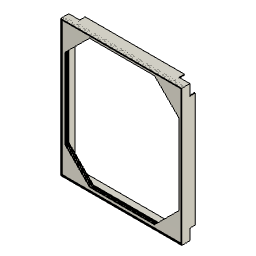
Step4-FaceFrame-4X (Autodesk Fusion 360 design; units mm, degrees)
Autodesk Fusion 360 part; units mm, degrees
note: some values were not read from the file. Set by a fixed rule: which sketch regions a step uses.
sketch "Sketch1" plane through (0, 0, 0) normal (0, 1, 0) x (1, 0, 0)
  line L0 (0, 0) -> (445, 0)
  line L1 (445, 0) -> (445, -500)
  line L2 (445, -500) -> (0, -500)
  line L3 (0, -500) -> (0, 0)
  dimension "d1" = 445
  dimension "d2" = 500
  constraint horizontal L0
  constraint vertical L1
  constraint horizontal L2
  constraint vertical L3
  constraint coincident L0.start L3.end
  measures "d1" distance of L0.start L0.end
  measures "d2" distance of L0.start L2.end
extrude "Extrude1" add sketch "Sketch1" along normal blind 50
ref_plane "WorkPlane1" through (222.5, 0, 250) normal (0, -1, 0) x (-1, 0, 0)
sketch "Sketch2" plane through (222.5, 0, 250) normal (0, -1, 0) x (1, 0, 0)
  line L0 (222.5, 250) -> (119.5, 250)
  line L1 (119.5, 250) -> (119.5, 237)
  line L2 (119.5, 237) -> (222.5, 237)
  line L3 (222.5, 237) -> (222.5, 250)
  line L4 (222.5, 250) -> (209.5, 250)
  line L5 (209.5, 250) -> (209.5, 147)
  line L6 (209.5, 147) -> (222.5, 147)
  line L7 (222.5, 147) -> (222.5, 250)
  line L8 (119.5, 237) -> (209.5, 147)
  line L9 (209.5, 237) -> (119.5, 237)
  line L10 (-222.5, 250) -> (-119.5, 250)
  line L11 (-119.5, 250) -> (-119.5, 237)
  line L12 (-119.5, 237) -> (-222.5, 237)
  line L13 (-222.5, 237) -> (-222.5, 250)
  line L14 (-222.5, 250) -> (-209.5, 250)
  line L15 (-209.5, 250) -> (-209.5, 147)
  line L16 (-209.5, 147) -> (-222.5, 147)
  line L17 (-222.5, 147) -> (-222.5, 250)
  line L18 (-222.5, -250) -> (-119.5, -250)
  line L19 (-119.5, -250) -> (-119.5, -237)
  line L20 (-119.5, -237) -> (-222.5, -237)
  line L21 (-222.5, -237) -> (-222.5, -250)
  line L22 (-222.5, -250) -> (-209.5, -250)
  line L23 (-209.5, -250) -> (-209.5, -147)
  line L24 (-209.5, -147) -> (-222.5, -147)
  line L25 (-222.5, -147) -> (-222.5, -250)
  line L26 (222.5, -250) -> (209.5, -250)
  line L27 (209.5, -250) -> (209.5, -147)
  line L28 (209.5, -147) -> (222.5, -147)
  line L29 (222.5, -147) -> (222.5, -250)
  line L30 (222.5, -250) -> (119.5, -250)
  line L31 (119.5, -250) -> (119.5, -237)
  line L32 (119.5, -237) -> (222.5, -237)
  line L33 (222.5, -237) -> (222.5, -250)
  line L34 (119.5, -237) -> (209.5, -147)
  line L35 (209.5, 147) -> (119.5, 237)
  line L36 (-119.5, 237) -> (-209.5, 147)
  line L37 (-209.5, -147) -> (-119.5, -237)
  line L38 (-209.5, 147) -> (-209.5, -147)
  line L39 (-119.5, -237) -> (119.5, -237)
  line L40 (209.5, 147) -> (209.5, -147)
  line L41 (119.5, 237) -> (-119.5, 237)
  dimension "d6" = 103
  dimension "d7" = 13
  dimension "d8" = 13
  dimension "d9" = 103
  dimension "d10" = 103
  dimension "d11" = 13
  dimension "d12" = 13
  dimension "d13" = 103
  dimension "d14" = 103
  dimension "d15" = 13
  dimension "d16" = 13
  dimension "d17" = 103
  dimension "d18" = 13
  dimension "d19" = 103
  dimension "d20" = 103
  dimension "d21" = 13
  constraint horizontal L0
  constraint vertical L1
  constraint horizontal L2
  constraint vertical L3
  constraint horizontal L4
  constraint vertical L5
  constraint horizontal L6
  constraint vertical L7
  constraint coincident L5 L9.start
  constraint coincident L2 L9.start
  constraint horizontal L10
  constraint vertical L11
  constraint horizontal L12
  constraint vertical L13
  constraint horizontal L14
  constraint vertical L15
  constraint horizontal L16
  constraint vertical L17
  constraint horizontal L18
  constraint vertical L19
  constraint horizontal L20
  constraint vertical L21
  constraint horizontal L22
  constraint vertical L23
  constraint horizontal L24
  constraint vertical L25
  constraint horizontal L26
  constraint vertical L27
  constraint horizontal L28
  constraint vertical L29
  constraint horizontal L30
  constraint vertical L31
  constraint horizontal L32
  constraint vertical L33
  constraint perpendicular L24 L38
  constraint perpendicular L31 L39
  constraint perpendicular L28 L40
  constraint perpendicular L11 L41
  measures "d6" distance of L0.start L0.end
  measures "d7" distance of L0.start L2.end
  measures "d8" distance of L0.start L4.end
  measures "d9" distance of L0.start L6.end
  measures "d10" distance of L10.start L10.end
  measures "d11" distance of L10.start L12.end
  measures "d12" distance of L10.start L14.end
  measures "d13" distance of L10.start L16.end
  measures "d14" distance of L18.start L18.end
  measures "d15" distance of L18.start L20.end
  measures "d16" distance of L18.start L22.end
  measures "d17" distance of L18.start L24.end
  measures "d18" distance of L26.start L26.end
  measures "d19" distance of L26.start L28.end
  measures "d20" distance of L26.start L30.end
  measures "d21" distance of L26.start L32.end
extrude "Extrude2" cut sketch "Sketch2" against normal blind 50 contours L8 L34 L35 L36 L37 L38 L39 L40 L41
ref_plane "WorkPlane2" through (442, 25, 250) normal (1, 0, 0) x (0, 0, -1)
sketch "Sketch3" plane through (442, 25, 250) normal (1, 0, 0) x (0, 1, 0)
  line L0 (-25, -250) -> (25, -250)
  line L1 (25, -250) -> (25, -247)
  line L2 (25, -247) -> (-25, -247)
  line L3 (-25, -247) -> (-25, -250)
  line L4 (-25, 250) -> (25, 250)
  line L5 (25, 250) -> (25, 247)
  line L6 (25, 247) -> (-25, 247)
  line L7 (-25, 247) -> (-25, 250)
  line L8 (-25, 247) -> (-22, 247)
  line L9 (-22, 247) -> (-22, -247)
  line L10 (-22, -247) -> (-25, -247)
  line L11 (-25, -247) -> (-25, 247)
  line L12 (-22, 247) -> (-19.4, 247)
  line L13 (-19.4, 247) -> (-19.4, 220.835)
  line L14 (-19.4, 220.835) -> (-22, 220.835)
  line L15 (-22, 220.835) -> (-22, 247)
  line L16 (-19.4, 247) -> (-16, 247)
  line L17 (-16, 247) -> (-16, -247)
  line L18 (-16, -247) -> (-19.4, -247)
  line L19 (-19.4, -247) -> (-19.4, 247)
  line L20 (-16, 247) -> (-13.4, 247)
  line L21 (-13.4, 247) -> (-13.4, 220.8212)
  line L22 (-13.4, 220.8212) -> (-16, 220.8212)
  line L23 (-16, 220.8212) -> (-16, 247)
  line L24 (-13.4, 247) -> (-10.4, 247)
  line L25 (-10.4, 247) -> (-10.4, -247)
  line L26 (-10.4, -247) -> (-13.4, -247)
  line L27 (-13.4, -247) -> (-13.4, 247)
  line L28 (-10.4, 247) -> (-7.8, 247)
  line L29 (-7.8, 247) -> (-7.8, 220.1918)
  line L30 (-7.8, 220.1918) -> (-10.4, 220.1918)
  line L31 (-10.4, 220.1918) -> (-10.4, 247)
  line L32 (-7.8, 247) -> (25, 247)
  line L33 (25, 247) -> (25, -247)
  line L34 (25, -247) -> (-7.8, -247)
  line L35 (-7.8, -247) -> (-7.8, 247)
  dimension "d25" = 3
  dimension "d26" = 50
  dimension "d27" = 3
  dimension "d28" = 3
  dimension "d29" = 2.6
  dimension "d30" = 3.4
  dimension "d31" = 2.6
  dimension "d32" = 3
  dimension "d33" = 2.6
  constraint horizontal L0
  constraint vertical L1
  constraint horizontal L2
  constraint vertical L3
  constraint horizontal L4
  constraint vertical L5
  constraint horizontal L6
  constraint vertical L7
  constraint horizontal L8
  constraint vertical L9
  constraint horizontal L10
  constraint vertical L11
  constraint horizontal L12
  constraint vertical L13
  constraint horizontal L14
  constraint vertical L15
  constraint horizontal L16
  constraint vertical L17
  constraint horizontal L18
  constraint vertical L19
  constraint horizontal L20
  constraint vertical L21
  constraint horizontal L22
  constraint vertical L23
  constraint horizontal L24
  constraint vertical L25
  constraint horizontal L26
  constraint vertical L27
  constraint horizontal L28
  constraint vertical L29
  constraint horizontal L30
  constraint vertical L31
  constraint horizontal L32
  constraint vertical L33
  constraint horizontal L34
  constraint vertical L35
  measures "d25" distance of L0.start L2.end
  measures "d26" distance of L4.start L4.end
  measures "d27" distance of L4.start L6.end
  measures "d28" distance of L6.end L8.end
  measures "d29" distance of L8.end L12.end
  measures "d30" distance of L12.end L16.end
  measures "d31" distance of L16.end L20.end
  measures "d32" distance of L20.end L24.end
  measures "d33" distance of L24.end L28.end
extrude "Extrude3" cut sketch "Sketch3" against normal blind 439 contours L2 L6 L8 L9 L10 L11 L15 | L2 L6 L29 L32 L33 L34 L35 | L2 L6 L13 L16 L17 L18 L19 L23 | L2 L6 L21 L24 L25 L26 L27 L31
ref_plane "WorkPlane3" through (222.5, 50, 250) normal (0, 1, 0) x (0, 0, 1)
sketch "Sketch4" plane through (222.5, 50, 250) normal (0, 1, 0) x (1, 0, 0)
  line L0 (222.5, -250) -> (182.5, -250)
  line L1 (182.5, -250) -> (182.5, -210)
  line L2 (182.5, -210) -> (222.5, -210)
  line L3 (222.5, -210) -> (222.5, -250)
  line L4 (-222.5, -250) -> (-182.5, -250)
  line L5 (-182.5, -250) -> (-182.5, -210)
  line L6 (-182.5, -210) -> (-222.5, -210)
  line L7 (-222.5, -210) -> (-222.5, -250)
  line L8 (-222.5, 250) -> (-182.5, 250)
  line L9 (-182.5, 250) -> (-182.5, 210)
  line L10 (-182.5, 210) -> (-222.5, 210)
  line L11 (-222.5, 210) -> (-222.5, 250)
  line L12 (222.5, 250) -> (182.5, 250)
  line L13 (182.5, 250) -> (182.5, 210)
  line L14 (182.5, 210) -> (222.5, 210)
  line L15 (222.5, 210) -> (222.5, 250)
  dimension "d37" = 40
  dimension "d38" = 40
  dimension "d39" = 40
  dimension "d40" = 40
  dimension "d41" = 40
  dimension "d42" = 40
  dimension "d43" = 40
  dimension "d44" = 40
  constraint horizontal L0
  constraint vertical L1
  constraint horizontal L2
  constraint vertical L3
  constraint horizontal L4
  constraint vertical L5
  constraint horizontal L6
  constraint vertical L7
  constraint horizontal L8
  constraint vertical L9
  constraint horizontal L10
  constraint vertical L11
  constraint horizontal L12
  constraint vertical L13
  constraint horizontal L14
  constraint vertical L15
  measures "d37" distance of L0.start L0.end
  measures "d38" distance of L0.start L2.end
  measures "d39" distance of L4.start L4.end
  measures "d40" distance of L4.start L6.end
  measures "d41" distance of L8.start L8.end
  measures "d42" distance of L8.start L10.end
  measures "d43" distance of L12.start L12.end
  measures "d44" distance of L12.start L14.end
extrude "Extrude4" cut sketch "Sketch4" against normal blind 20
ref_plane "WorkPlane4" through (425, 30, 20) normal (0, 1, 0) x (0, 0, 1)
sketch "Sketch5" plane through (425, 30, 20) normal (0, 1, 0) x (1, 0, 0)
  line L0 (20, 20) -> (-20, 20)
  line L1 (-20, 20) -> (-20, -20)
  line L2 (-20, -20) -> (20, -20)
  line L3 (20, -20) -> (20, 20)
  line L4 (-425, 20) -> (-385, 20)
  line L5 (-385, 20) -> (-385, -20)
  line L6 (-385, -20) -> (-425, -20)
  line L7 (-425, -20) -> (-425, 20)
  line L8 (-425, -480) -> (-385, -480)
  line L9 (-385, -480) -> (-385, -440)
  line L10 (-385, -440) -> (-425, -440)
  line L11 (-425, -440) -> (-425, -480)
  line L12 (20, -480) -> (-20, -480)
  line L13 (-20, -480) -> (-20, -440)
  line L14 (-20, -440) -> (20, -440)
  line L15 (20, -440) -> (20, -480)
  dimension "d48" = 40
  dimension "d49" = 40
  dimension "d50" = 40
  dimension "d51" = 40
  dimension "d52" = 40
  dimension "d53" = 40
  dimension "d54" = 40
  dimension "d55" = 40
  constraint horizontal L0
  constraint vertical L1
  constraint horizontal L2
  constraint vertical L3
  constraint horizontal L4
  constraint vertical L5
  constraint horizontal L6
  constraint vertical L7
  constraint horizontal L8
  constraint vertical L9
  constraint horizontal L10
  constraint vertical L11
  constraint horizontal L12
  constraint vertical L13
  constraint horizontal L14
  constraint vertical L15
  measures "d48" distance of L0.start L0.end
  measures "d49" distance of L0.start L2.end
  measures "d50" distance of L4.start L4.end
  measures "d51" distance of L4.start L6.end
  measures "d52" distance of L8.start L8.end
  measures "d53" distance of L8.start L10.end
  measures "d54" distance of L12.start L12.end
  measures "d55" distance of L12.start L14.end
extrude "Extrude5" add sketch "Sketch5" against normal blind 13
ref_plane "WorkPlane5" through (222.5, 3, 250) normal (0, -1, 0) x (0, 0, 1)
sketch "Sketch6" plane through (222.5, 3, 250) normal (0, -1, 0) x (1, 0, 0)
ref_plane "WorkPlane6" through (425, 30, 480) normal (0, 1, 0) x (0, 0, 1)
sketch "Sketch7" plane through (425, 30, 480) normal (0, 1, 0) x (1, 0, 0)
  line L0 (20, -20) -> (0, -20)
  line L1 (0, -20) -> (0, 0)
  line L2 (0, 0) -> (20, 0)
  line L3 (20, 0) -> (20, -20)
  circle A0 centre (0, 0) radius 7.5
  line L4 (-425, -20) -> (-405, -20)
  line L5 (-405, -20) -> (-405, 0)
  line L6 (-405, 0) -> (-425, 0)
  line L7 (-425, 0) -> (-425, -20)
  circle A1 centre (-405, 0) radius 7.5
  line L8 (-425, 480) -> (-405, 480)
  line L9 (-405, 480) -> (-405, 460)
  line L10 (-405, 460) -> (-425, 460)
  line L11 (-425, 460) -> (-425, 480)
  circle A2 centre (-405, 460) radius 7.5
  line L12 (20, 480) -> (0, 480)
  line L13 (0, 480) -> (0, 460)
  line L14 (0, 460) -> (20, 460)
  line L15 (20, 460) -> (20, 480)
  circle A3 centre (0, 460) radius 7.5
  dimension "d60" = 20
  dimension "d61" = 20
  dimension "d62" = 15
  dimension "d63" = 20
  dimension "d64" = 20
  dimension "d65" = 15
  dimension "d66" = 20
  dimension "d67" = 20
  dimension "d68" = 15
  dimension "d69" = 20
  dimension "d70" = 20
  dimension "d71" = 15
  constraint horizontal L0
  constraint vertical L1
  constraint horizontal L2
  constraint vertical L3
  constraint coincident L1.end L2.start
  constraint horizontal L4
  constraint vertical L5
  constraint horizontal L6
  constraint vertical L7
  constraint coincident L5.end L6.start
  constraint horizontal L8
  constraint vertical L9
  constraint horizontal L10
  constraint vertical L11
  constraint coincident L9.end L10.start
  constraint horizontal L12
  constraint vertical L13
  constraint horizontal L14
  constraint vertical L15
  constraint coincident L13.end L14.start
  measures "d60" distance of L0.start L0.end
  measures "d61" distance of L0.start L2.end
  measures "d62" diameter of A0
  measures "d63" distance of L4.start L4.end
  measures "d64" distance of L4.start L6.end
  measures "d65" diameter of A1
  measures "d66" distance of L8.start L8.end
  measures "d67" distance of L8.start L10.end
  measures "d68" diameter of A2
  measures "d69" distance of L12.start L12.end
  measures "d70" distance of L12.start L14.end
  measures "d71" diameter of A3
extrude "Extrude6" cut sketch "Sketch7" against normal blind 2.65 contours L1 L2 A0 | L1 L2 A0 | L5 L6 A1 | L5 L6 A1 | L9 L10 A2 | L9 L10 A2 | L13 L14 A3 | L13 L14 A3
